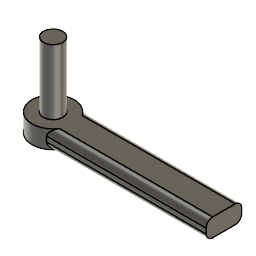
Slider & Revolute joint (Autodesk Fusion 360 design; units mm, degrees)
Autodesk Fusion 360 part; units mm, degrees
sketch "Sketch1" plane through (0, 0, 0) normal (0, 0, 1) x (1, 0, 0)
  line L0 (1.7321, 2.75) -> (26.3431, 2.75)
  line L1 (26.3431, 2.75) -> (26.3431, -2.75)
  line L2 (26.3431, -2.75) -> (1.7321, -2.75)
  arc A0 (1.7321, 2.75) -> (1.7321, -2.75) centre (0, 0) ccw
  dimension "d1" = 6.5
  dimension "d2" = 5.5
  dimension "d3" = 24.611
  dimension "d4" = 5.5
  constraint coincident A0.centre origin
  constraint perpendicular L0 L1
  measures "d1" diameter of A0
  measures "d2" distance of L0.start L2.end
  measures "d3" distance of L0.start L0.end
  measures "d4" distance of L0.end L1.end
sketch "Sketch2" plane through (0, 0, 0) normal (0, 0, 1) x (1, 0, 0)
sketch "Sketch3" plane through (0, 0, 0) normal (0, 0, 1) x (1, 0, 0)
extrude "Extrude1" add sketch "Sketch1" along normal blind 2.8
sketch "Sketch4" plane through (0, 0, 2.8) normal (0, 0, 1) x (-1, 0, 0)
  line L0 (-26.3431, -2.75) -> (-1.7321, -2.75)
  arc A0 (-1.7321, -2.75) -> (-1.7321, 2.75) centre (0, 0) ccw
  line L1 (-1.7321, 2.75) -> (-26.3431, 2.75)
  line L2 (-26.3431, 2.75) -> (-26.3431, -2.75)
  circle A1 centre (0, 0) radius 1.5
  dimension "d7" = 3
  constraint concentric A0 A1
  measures "d7" diameter of A1
extrude "Extrude2" add sketch "Sketch4" along normal blind 10 contours A1
fillet "Fillet1" radius 1 4 edges at (14.0376, -2.75, 2.8) (14.0376, 2.75, 2.8) (14.0376, 2.75, 0) (14.0376, -2.75, 0)
